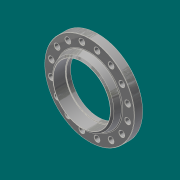
# Autodesk Inventor part: A1-19027-400-06 Alco flange - 12in CL300
Saved by Autodesk Inventor 2017.3 (Build 213257000, 257)
## iProperties
Created: 2019-06-24
Part Number: A1-19027-400-06 Alco flange - 12in CL300
Material: Steel, Mild
Document SubType Name: Modeling
Designer: Graeme_Van_Dongen
Density: 7.85 g/cm^3
Appearance: Steel
Mass: 51776.7 g
Surface Area: 5235.02 cm^2
Volume: 6595.76 cm^3
Description: 12" CLASS 300 RF ALCO FLANGE, A350 LF2, Ø12 5/8" BORE, MATES TO B16.5 CLASS 300
Author: Graeme_Van_Dongen
Autodesk Inventor part; units mm, degrees
ref_plane "YZ Plane" through (0, 0, 0) normal (1, 0, 0) x (0, 1, 0)
ref_plane "XZ Plane" through (0, 0, 0) normal (0, 1, 0) x (-1, 0, 0)
ref_plane "XY Plane" through (0, 0, 0) normal (0, 0, 1) x (1, 0, 0)
sketch "Sketch1" plane through (0, 0, 0) normal (1, 0, 0) x (0, 1, 0)
  line L0 (0, 0) -> (0, 95.25)
  line L1 (190.5, 0) -> (165.1, 0)
  line L2 (165.1, 0) -> (165.1, 95.25)
  line L3 (165.1, 95.25) -> (166.6875, 95.25)
  line L4 (166.6875, 95.25) -> (177.8, 86.7231)
  line L5 (177.8, 86.7231) -> (188.1037, 54.3397)
  arc A0 (188.1037, 54.3397) -> (192.9446, 50.8) centre (192.9446, 55.88) ccw
  line L6 (192.9446, 50.8) -> (260.35, 50.8)
  line L7 (260.35, 50.8) -> (260.35, 1.5875)
  line L8 (260.35, 1.5875) -> (190.5, 1.5875)
  line L9 (190.5, 1.5875) -> (190.5, 0)
  point P0 (189.23, 50.8)
  dimension "d0" = 95.25
  dimension "d1" = 520.7
  dimension "d2" = 50.8
  dimension "d3" = 381
  dimension "d4" = 1.5875
  dimension "d5" = 355.6
  dimension "d6" = 330.2
  dimension "d7" = 378.46
  dimension "d8" = 37.5
  dimension "d9" = 11.1125
  dimension "d10" = 5.08
  constraints: 20 end point, 5 perpendicular, 4 point on line, 2 point on circle, 2 tangent, 1 centre point, 1 horizontal, 1 parallel, 1 vertical
  measures "d0" distance of L0.start L0.end
  measures "d1" diameter of L7 L0
  measures "d2" distance between parallel lines of L6 L1
  measures "d3" diameter of L9 L0
  measures "d4" distance between parallel lines of L8 L1
  measures "d5" diameter of L4.end L0
  measures "d6" diameter of L2 L0
  measures "d7" diameter of point (189.23, 50.8) L0
  measures "d8" angle of L3 L4
  measures "d9" horizontal distance of L3.end L4.end
  measures "d10" radius of A0
revolve "Revolution1" add sketch "Sketch1" angle 360 about axis through (0, 0, 0) along (0, 0, 1)
sketch "Sketch2" plane through (0, 0, 50.8) normal (0, 0, 1) x (1, 0, 0)
  line L0 (0, -364.49) -> (0, 364.49) construction
  line L1 (-43.9782, -221.0935) -> (43.9782, 221.0935) construction
  point P0 (0, 0)
  dimension "d12" = 450.85
  dimension "d13" = 11.25
  constraints: 2 end point, 1 coincident, 1 midpoint
  measures "d12" distance of L1.start L1.end
  measures "d13" angle of L0 L1
hole "Hole1" at (43.9782, 221.0935, 50.8) direction (0, 0, -1) diameter 31.75 end through all
chamfer "Chamfer1" distance 1.5875 angle 45 2 edges at (43.9782, 236.9685, 50.8) (43.9782, 236.9685, 1.5875)
pattern_circular "Circular Pattern1" count 16 over 360 about axis through (0, 0, -10) along (0, 0, 1) of "Hole1", "Chamfer1"
chamfer "Chamfer2" distance 1.5875 angle 45 2 edges at (0, -260.35, 50.8) (0, -260.35, 1.5875)
sketch "Sketch3" plane through (0, 0, 0) normal (0, 0, -1) x (-1, 0, 0)
  circle A0 centre (0, 0) radius 165.1 projected
  circle A1 centre (0, 0) radius 160.3375
  dimension "d30" = 320.675
  constraints: 1 centre point, 1 coincident
  measures "d30" diameter of A1
extrude "Extrusion1" add sketch "Sketch3" against normal blind 25.4
fillet "Fillet1" radius 0.7937 1 edges at (0, -165.1, 25.4)
chamfer "Chamfer3" distance 0.7937 angle 45 1 edges at (160.3375, 0, 25.4)
equation "\"d0\" = Length"
equation "\"d1\" = OutsideDiameter"
equation "\"d2\" = Thickness"
equation "\"d3\" = RFDiameter"
equation "\"d4\" = RFThickness"
equation "\"d5\" = CasingDiameter"
equation "\"d6\" = Bore"
equation "\"d7\" = HubDiameter"
equation "\"d8\" = WeldBevelAngle"
equation "\"d9\" = WeldBevelSize"
equation "\"d10\" = HubRadius"
equation "\"d12\" = BCD"
equation "\"d14\" = HoleDiameter"
equation "\"d21\" = HoleChamfer"
equation "\"d27\" = RimChamfer"
equation "\"OutsideDiameter\" = 520.7"
equation "\"Thickness\" = 50.8"
equation "\"Length\" = 95.25"
equation "\"RFDiameter\" = 381"
equation "\"CasingDiameter\" = 355.6"
equation "\"Bore\" = 330.2"
equation "\"HoleDiameter\" = 31.75"
equation "\"BCD\" = 450.85"
equation "\"RFThickness\" = 1.5875"
equation "\"WeldBevelAngle\" = 37.5deg"
equation "\"HubDiameter\" = 378.46"
equation "\"HoleChamfer\" = 1.5875"
equation "\"RimChamfer\" = 1.5875"
equation "\"HubRadius\" = 5.08"
equation "\"WeldBevelSize\" = 11.1125"
body "Solid1"
